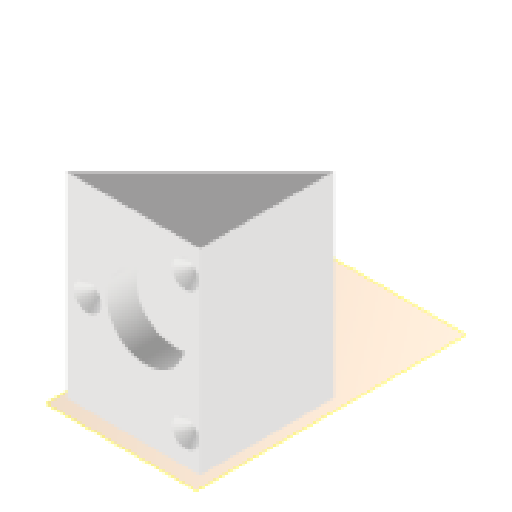
# Autodesk Inventor part: TIRFImager_KinematicMirror_v3
Saved by Autodesk Inventor 2024.1 (Build 281209000, 209)
## iProperties
Created: 2024-07-28
Part Number: TIRFImager_KinematicMirror_v3
Material: Generisch
Document SubType Name: Modeling
Designer: diederichbenedict
Density: 1 g/cm^3
Appearance: Vorgabe
Author: diederichbenedict
Autodesk Inventor part; units mm, degrees
ref_plane "YZ Plane" through (0, 0, 0) normal (1, 0, 0) x (0, 1, 0)
ref_plane "XZ Plane" through (0, 0, 0) normal (0, 1, 0) x (-1, 0, 0)
ref_plane "XY Plane" through (0, 0, 0) normal (0, 0, 1) x (1, 0, 0)
ref_plane "Arbeitsebene1" through (0, 0, 1) normal (0, 0, 1) x (1, 0, 0)
sketch "Skizze1" plane through (0, 0, 1) normal (0, 0, 1) x (1, 0, 0)
  line L0 (0, -25) -> (0, 0) projected
  line L1 (0, -25) -> (14, -25) projected
  line L2 (14, 0) -> (14, -25) projected
  line L3 (0, 0) -> (14, 0) projected
  line L4 (-1, -11.3514) -> (-6.5, -11.3514) construction
  line L5 (-4.5, -14.125) -> (-37.3, -14.125) construction
  line L6 (-1, -16.6486) -> (-6.5, -16.6486) construction
  line L7 (4, 20.8392) -> (4, 0) construction
  line L8 (12, 20.8392) -> (12, 0) construction
  line L9 (8, 20.6561) -> (8, -14) construction
  line L10 (-4.5, -14) -> (8, -14) construction
  line L11 (1.6137, -20.3863) -> (12.8954, -9.1046) construction
  line L12 (1.6137, -20.3863) -> (17.5684, -20.3863) construction
  line L13 (0, -25) -> (14, -25) construction
  line L14 (0, -24.6915) -> (13.5, -24.6915)
  line L15 (13.5, -24.6915) -> (13.5, -11.0456)
  line L16 (13.5, -11.0456) -> (0, -24.5456)
  line L17 (0, -24.6915) -> (0, -24.5456)
  dimension "d0" = 4
  dimension "d1" = 5.2972
  dimension "d2" = 2.6486
  dimension "d3" = 45
  dimension "d4" = 1.8
  dimension "d5" = 0.5
  constraints: 24 end point, 5 horizontal, 3 point on line, 3 vertical, 1 collinear, 1 equal length, 1 parallel, 1 perpendicular, 8 other
  measures "d0" distance between parallel lines of L7 L9
  measures "d1" distance between parallel lines of L6 L4
  measures "d2" distance between parallel lines of L4 L10
  measures "d3" angle of L12 L11
  measures "d4" distance between parallel lines of L16 L11
  measures "d5" distance between parallel lines of L2 L15
extrude "Extrusion1" add sketch "Skizze1" along normal blind 20 contours L0 L16 L15 L14
sketch "Skizze2" plane through (0, -24.6915, 1) normal (0, -1, 0) x (1, 0, 0)
  circle A0 centre (12, 17) radius 1.4 projected
  line L0 (0, 2.559) -> (10.6713, 2.559) projected
  circle A1 centre (12, 3) radius 1.4 projected
  circle A2 centre (2, 10) radius 1.4 projected
  point P0 (0, -1)
  constraints: 1 other
hole "Bohrung1" at (12, -24.6915, 18) at (12, -24.6915, 4) at (2, -24.6915, 11) direction (0, 1, 0) diameter 2.8 depth 0.001 tip angle 80
sketch "Skizze3" plane through (0, -24.6915, 1) normal (0, -1, 0) x (1, 0, 0)
  line L0 (0, 20) -> (13.5, 20) projected
  line L1 (0, 0) -> (13.5, 0) projected
  line L2 (13.5, 0) -> (13.5, 20) projected
  line L3 (0, -7) -> (0, 29) projected
  circle A0 centre (7.9714, 11) radius 4
  point P0 (0, -1)
  dimension "d15" = 8
  constraints: 1 centre point
  measures "d15" diameter of A0
extrude "Extrusion2" cut sketch "Skizze3" against normal blind 3 contours A0
equation "\"d2\" = 0.5 * d1"
